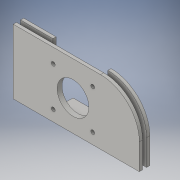
# Autodesk Inventor part: RemoteExtruderV4
Saved by Autodesk Inventor 2016 (Build 200138000, 138)
## iProperties
Created: 2016-02-22
Part Number: RemoteExtruderV4
Material: Generic
Document SubType Name: Modeling
Designer: Scott
Density: 1 g/cm^3
Appearance: Default
Author: Scott
Autodesk Inventor part; units mm, degrees
ref_plane "YZ Plane" through (0, 0, 0) normal (1, 0, 0) x (0, 1, 0)
ref_plane "XZ Plane" through (0, 0, 0) normal (0, 1, 0) x (-1, 0, 0)
ref_plane "XY Plane" through (0, 0, 0) normal (0, 0, 1) x (1, 0, 0)
sketch "Sketch1" plane through (0, 0, 0) normal (0, 0, 1) x (1, 0, 0)
  circle A0 centre (0, 0) radius 12.5
  line L0 (0, 0) -> (15.5, 0)
  line L1 (0, 0) -> (15.5, 0) construction
  line L2 (15.5, 0) -> (15.5, 15.5)
  circle A1 centre (15.5, 15.5) radius 1.5
  circle A2 centre (-15.5, 15.5) radius 1.5
  circle A3 centre (15.5, -15.5) radius 1.5
  circle A4 centre (-15.5, -15.5) radius 1.5
  line L3 (21.59, -21.59) -> (-21.59, -21.59)
  line L4 (-21.59, -21.59) -> (-21.59, 21.59)
  line L5 (-21.59, 21.59) -> (21.59, 21.59)
  line L6 (21.59, 21.59) -> (21.59, -21.59)
  line L7 (21.59, -21.59) -> (-21.59, 21.59) construction
  line L8 (-21.59, -21.59) -> (21.59, 21.59) construction
  dimension "d0" = 25
  dimension "d1" = 15.5
  dimension "d2" = 0
  dimension "d3" = 15.5
  dimension "d4" = 3
  dimension "d7" = 31
  dimension "d10" = 31
  dimension "d13" = 43.18
  dimension "d14" = 43.18
  constraints: 18 end point, 5 centre point, 4 horizontal, 2 coincident, 2 midpoint, 2 parallel, 2 perpendicular, 1 collinear, 1 vertical, 6 other
  measures "d0" diameter of A0
  measures "d1" distance of L0.start L0.end
  measures "d2" distance between parallel lines of L0 L1
  measures "d3" distance of L0.end L2.end
  measures "d4" diameter of A1
  measures "d7" distance of A1.centre A2.centre
  measures "d10" distance of A1.centre A3.centre
  measures "d13" distance of L4.end L5.end
  measures "d14" distance of L3.end L4.end
extrude "Extrusion1" add sketch "Sketch1" along normal blind 3.81
sketch "Sketch2" plane through (-21.59, -21.59, 0) normal (0, -1, 0) x (1, 0, 0)
  line L0 (0, 3.81) -> (43.18, 3.81) projected
  line L1 (0, 3.81) -> (43.18, 3.81)
  line L2 (43.18, 3.81) -> (43.18, -17.78)
  line L3 (43.18, -17.78) -> (0, -17.78)
  line L4 (0, -17.78) -> (0, 3.81)
  point P0 (21.59, 0)
  dimension "d17" = 21.59
  constraints: 8 end point, 2 parallel, 1 horizontal, 1 perpendicular
  measures "d17" distance of L1.end L2.end
extrude "Extrusion2" add sketch "Sketch2" along normal blind 2.54
sketch "Sketch3" plane through (0, 0, 3.81) normal (0, 0, 1) x (1, 0, 0)
  line L0 (-21.59, 21.59) -> (21.59, 21.59) projected
  circle A0 centre (0, 0) radius 12.5 projected
  circle A1 centre (-15.5, -15.5) radius 1.5 projected
  circle A2 centre (15.5, -15.5) radius 1.5 projected
  circle A3 centre (-15.5, 15.5) radius 1.5 projected
  circle A4 centre (15.5, 15.5) radius 1.5 projected
  line L1 (21.59, 21.59) -> (21.59, -24.13) projected
  line L2 (21.59, 21.59) -> (-21.59, 21.59) projected
  line L3 (-21.59, 21.59) -> (-21.59, -24.13) projected
  line L4 (21.59, -24.13) -> (-21.59, -24.13) projected
  line L5 (-21.59, 26.67) -> (21.59, 26.67)
  arc A5 (52.07, -3.81) -> (21.59, 26.67) centre (21.59, -3.81) ccw
  line L6 (52.07, -3.81) -> (52.07, -24.13)
  line L7 (-21.59, 26.67) -> (-21.59, 21.59)
  line L8 (-21.59, 21.59) -> (21.59, 21.59)
  line L9 (21.59, 21.59) -> (21.59, -21.59) projected
  line L10 (21.59, 21.59) -> (21.59, -24.13)
  line L11 (21.59, 21.59) -> (21.59, -24.13) projected
  line L12 (21.59, -24.13) -> (52.07, -24.13)
  constraints: 12 end point, 2 collinear, 2 point on circle, 1 centre point, 1 perpendicular, 1 vertical
extrude "Extrusion3" add sketch "Sketch3" against normal blind 2.54 contours L7 L5 A5 L6 L12 L1 L0
sketch "Sketch4" plane through (0, 0, 1.27) normal (0, 0, -1) x (-1, 0, 0)
  line L0 (-21.59, 21.59) -> (-21.59, -24.13) projected
  line L1 (-21.59, -24.13) -> (-46.99, -24.13)
  arc A0 (-21.59, 26.67) -> (-52.07, -3.81) centre (-21.59, -3.81) ccw projected
  arc A1 (-21.59, 21.59) -> (-46.99, -3.81) centre (-21.59, -3.81) ccw
  line L2 (-46.99, -3.81) -> (-46.99, -24.13)
  line L3 (-21.59, 21.59) -> (-21.59, -24.13)
  line L4 (-21.59, 21.59) -> (-21.59, -24.13)
  line L5 (-21.59, -24.13) -> (-21.59, 21.59)
  point P0 (0, 0)
  dimension "d26" = 25.4
  dimension "d27" = 5.08
  constraints: 10 end point, 2 collinear, 2 point on circle, 1 centre point, 1 vertical
  measures "d26" distance of L0.end L1.end
  measures "d27" radial gap between concentric circles of A0 A1
extrude "Extrusion4" add sketch "Sketch4" along normal blind 3.175
sketch "Sketch5" plane through (0, 0, -1.905) normal (0, 0, -1) x (-1, 0, 0)
  line L0 (-46.99, -24.13) -> (-46.99, -3.81) projected
  arc A0 (-21.59, 21.59) -> (-46.99, -3.81) centre (-21.59, -3.81) ccw projected
  line L1 (21.59, 21.59) -> (-21.59, 21.59) projected
  line L2 (21.59, 21.59) -> (21.59, 26.67) projected
  line L3 (21.59, 26.67) -> (-21.59, 26.67) projected
  arc A1 (-21.59, 26.67) -> (-52.07, -3.81) centre (-21.59, -3.81) ccw projected
  line L4 (-52.07, -3.81) -> (-52.07, -24.13) projected
  line L5 (-52.07, -24.13) -> (-46.99, -24.13) projected
  line L6 (-21.59, -21.59) -> (-21.59, -24.13) projected
  line L7 (-21.59, -21.59) -> (-21.59, 21.59) projected
  arc A2 (-21.59, 21.59) -> (-46.99, -3.81) centre (-21.59, -3.81) ccw projected
  line L8 (-46.99, -3.81) -> (-46.99, -24.13) projected
  line L9 (-46.99, -24.13) -> (-21.59, -24.13) projected
  line L10 (21.59, 21.59) -> (-21.59, 21.59) projected
  line L11 (-21.59, 21.59) -> (-21.59, 26.67)
  point P0 (0, 0)
  constraints: 2 end point, 1 perpendicular
extrude "Extrusion5" add sketch "Sketch5" along normal blind 2.54 contours L5 L4 A1 L11 A0 L0 | L0 A0 L7 L6 L9
sketch "Sketch6" plane through (-21.59, -21.59, 0) normal (-1, 0, 0) x (0, 0, 1)
  line L0 (0, 43.18) -> (0, 0) projected
  line L1 (0, 43.18) -> (-1.905, 43.18) projected
  line L2 (-1.905, 43.18) -> (-1.905, 48.26) projected
  line L3 (-1.905, 48.26) -> (-4.445, 48.26) projected
  line L4 (-4.445, 0) -> (-4.445, 48.26) projected
  line L5 (0, 0) -> (-4.445, 0) projected
  line L6 (1.27, 17.78) -> (1.27, 43.18) projected
  line L7 (0, 0) -> (0, 43.18) projected
  line L8 (-17.78, 0) -> (0, 0) projected
  line L9 (-17.78, 0) -> (-17.78, -2.54) projected
  line L10 (3.81, -2.54) -> (-17.78, -2.54) projected
  line L11 (3.81, 48.26) -> (3.81, -2.54) projected
  line L12 (3.81, 48.26) -> (1.27, 48.26) projected
  line L13 (1.27, 43.18) -> (1.27, 48.26) projected
  line L14 (0, 43.18) -> (1.27, 43.18) projected
  line L15 (-4.445, 0) -> (-17.78, 0) projected
  line L16 (-17.78, -2.54) -> (-4.445, -2.54) projected
  line L17 (-4.445, 0) -> (-4.445, -2.54)
  point P0 (0, 21.59)
  constraints: 2 end point, 1 vertical
extrude "Extrusion6" add sketch "Sketch6" along normal blind 25.4 contours L14 L13 L12 L11 L10 L17 L5 L0 | L0 L5 L4 L3 L2 L1
body "Solid1"
